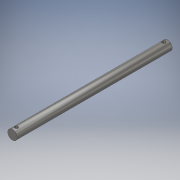
# Autodesk Inventor part: VS-007 (HANDLE ROD)
Saved by Autodesk Inventor 2017 (Build 210142000, 142)
## iProperties
Created: 2016-12-05
Part Number: VS-007 (HANDLE ROD)
Material: Steel, Alloy
Document SubType Name: Modeling
Designer: OCCC
Density: 7.73 g/cm^3
Appearance: Semi-Polished
Author: OCCC
Autodesk Inventor part; units mm, degrees
ref_plane "YZ Plane" through (0, 0, 0) normal (1, 0, 0) x (0, 1, 0)
ref_plane "XZ Plane" through (0, 0, 0) normal (0, 1, 0) x (-1, 0, 0)
ref_plane "XY Plane" through (0, 0, 0) normal (0, 0, 1) x (1, 0, 0)
sketch "Sketch1" plane through (0, 0, 0) normal (0, 0, 1) x (1, 0, 0)
  circle A0 centre (0, 0) radius 3.956
  dimension "d0" = 7.9121
  constraints: 1 centre point, 1 coincident
  measures "d0" diameter of A0
extrude "Extrusion1" add sketch "Sketch1" against normal blind 130.175
sketch "Sketch2" plane through (0, 0, 0) normal (0, 1, 0) x (-1, 0, 0)
  circle A0 centre (0, -3.175) radius 1.3208
  circle A1 centre (0, -127) radius 1.3208
  line L0 (-3.956, 0) -> (3.956, 0) projected
  line L1 (-3.956, -130.175) -> (3.956, -130.175) projected
  point P0 (0, 0)
  dimension "d3" = 2.6416
  dimension "d4" = 2.6416
  dimension "d5" = 3.175
  dimension "d6" = 3.175
  constraints: 2 centre point, 2 vertical alignment
  measures "d3" diameter of A1
  measures "d4" diameter of A0
  measures "d5" distance from line of A0.centre L0
  measures "d6" distance from line of L1 A1.centre
extrude "Extrusion2" cut sketch "Sketch2" along normal through all both and the other way through all
body "Solid1"
